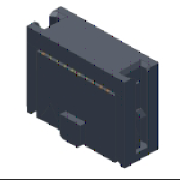
# Autodesk Inventor part: Ribbon Cable Connector-02
Saved by Autodesk Inventor 2017 (Build 210142000, 142)
## iProperties
Created: 2016-02-22
Part Number: Ribbon Cable Connector-02
Material: Generic
Description: 2.54mm (0.10in) Pitch, Receptacle, Vertical, Dual Row
Document SubType Name: Modeling
Designer: qupec
Language: en-US
Size Designation: Ribbon Cable Connector-01
Categories: <MemberInstance><Categories><Category DisplayName="Cable &amp; Harness" InternalName="e4a7e005-5e42-4d16-b293-125e7f0d0512" Mnemonic="CABLEANDHARNESS"><Category DisplayName="Connectors" InternalName="6f634eba-a678-4820-a31d-2c2d5ee6728e" Mnemonic="CONNECTORS"><CategoryParameter DisplayName="RefDes" InternalName="c3740e8c-60ab-4d5d-8584-52b73222f2f0" Mnemonic="REFDES"/><Category DisplayName="Ribbon Cable" InternalName="27621a3d-53ec-49ed-8225-e2ac65e8eb52" Mnemonic="RIBBONCABLE"/></Category></Category><Category DisplayName="DataType" InternalName="23b78d0f-2648-40c6-8793-ca6db495c9e8" Mnemonic="DATATYPE"><CategoryParameter DisplayName="DisplayName" InternalName="05415f3d-3907-474b-a020-eb9d644f4cf3" Mnemonic="DISPLAYNAME"/><CategoryParameter DisplayName="Standard" InternalName="0c0a119c-1e12-4c84-803f-101930972f5e" Mnemonic="STANDARD"/><CategoryParameter DisplayName="Description" InternalName="13903e3d-64b1-4950-80da-f627842ea37f" Mnemonic="DESCRIPTION"/><CategoryParameter DisplayName="Designation" InternalName="2675968c-4ce5-49e0-a4f5-552d29089031" Mnemonic="DESIGNATION"/><CategoryParameter DisplayName="Default Row" InternalName="2af9ec52-faaa-4026-b378-f9fa4afca842" Mnemonic="DEFAULTROW"/><CategoryParameter DisplayName="Folder Name" InternalName="3f06958e-8713-4116-9be7-ed6184ecc97b" Mnemonic="FOLDERNAME"/><CategoryParameter DisplayName="Revision Guid" InternalName="45a75005-10b1-4dfc-8d6d-dfe629f0b93c" Mnemonic="REVISIONGUID"/><CategoryParameter DisplayName="FileName" InternalName="8b46a4cc-9585-4fed-90c3-899f57e09a73" Mnemonic="FILENAME"/><CategoryParameter DisplayName="StdsOrg" InternalName="8f5914e1-4693-403f-8ab5-d37768198c9d" Mnemonic="STDSORG"/><CategoryParameter DisplayName="Family Version" InternalName="914462f6-6e19-4b14-ba84-155b9680b1d0" Mnemonic="FAMILYREVISION"/><CategoryParameter DisplayName="Standard Revision" InternalName="91d5a463-65c2-4fde-b823-3b7fea5e8e17" Mnemonic="STANDARDREVISION"/><CategoryParameter DisplayName="Member Revision" InternalName="a65d44b9-392f-4f4f-857b-e4b3d54996fe" Mnemonic="MEMBERREVISION"/><CategoryParameter DisplayName="ClipFormat" InternalName="bc51e27b-3422-4e78-93ef-cec197ddf230" Mnemonic="CLIPFORMAT"/><CategoryParameter DisplayName="Manufacturer" InternalName="cd6c7a72-a28a-4e50-99a9-2c7f4e13e5ad" Mnemonic="MANUFACTURER"/><CategoryParameter DisplayName="InternalName" InternalName="cf1d0246-76d9-4b4a-8305-fa0409afb5c1" Mnemonic="INTERNALNAME"/><CategoryParameter DisplayName="IsMetric" InternalName="e2385c5b-1ea4-4823-96a8-8de651266ec3" Mnemonic="ISMETRIC"/><Category DisplayName="Part" InternalName="c0e0b642-3bcb-4cc8-9e80-f96d35c4afa4" Mnemonic="PART"><CategoryParameter DisplayName="Part Number" InternalName="016b6077-bfbe-49bd-92c9-d8d59c39c941" Mnemonic="PARTNUMBER"/><CategoryParameter DisplayName="Stock Number" InternalName="4dba7c1c-e26c-444e-836c-b08b433409a8" Mnemonic="STOCKNUMBER"/><CategoryParameter DisplayName="Material Key" InternalName="5c9a8adb-dd2b-4535-b97f-0a94a95fe41f" Mnemonic="MATERIALKEY"/><CategoryParameter DisplayName="Material" InternalName="818a152a-d3c3-49ca-80ee-df7d91421b8e" Mnemonic="MATERIAL"/></Category></Category></Categories><FamilyTemplate Id="Ribbon Cable Connector"><FamilyTemplateParameters><FamilyTemplateParameter ObjectType="kUserParameterObject" ValueType="xs:double" Id="1" ObjectReferenceKey="Circuits"/><FamilyTemplateParameter ObjectType="kUserParameterObject" ValueType="xs:double" Id="2" ObjectReferenceKey="DimA"/><FamilyTemplateParameter ObjectType="kUserParameterObject" ValueType="xs:double" Id="3" ObjectReferenceKey="DimB"/><FamilyTemplateParameter ObjectType="kPropertyObject" ValueType="xs:string" Id="100" ObjectReferenceKey="{32853F0F-3444-11d1-9E93-0060B03C1CA6}" SubObjectId="52"/><FamilyTemplateParameter ObjectType="kPropertyObject" ValueType="xs:string" Id="105" ObjectReferenceKey="{32853F0F-3444-11d1-9E93-0060B03C1CA6}" SubObjectId="5"/><FamilyTemplateParameter ObjectType="kPartComponentDefinitionObject" ValueType="xs:string" Id="110" SubObjectId="Material"/><FamilyTemplateParameter ObjectType="kPartFeatureObject" ValueType="xs:boolean" Id="200" ObjectReferenceKey="1002000010000000700a0100000000008000000000000000" SubObjectId="Suppressed"/><FamilyTemplateParameter ObjectType="kPartFeatureObject" ValueType="xs:boolean" Id="201" ObjectReferenceKey="1002000010000000320b0100000000008000000000000000" SubObjectId="Suppressed"/><FamilyTemplateParameter ObjectType="kPartFeatureObject" ValueType="xs:boolean" Id="202" ObjectReferenceKey="100200001000000044680200000000008000000000000000" SubObjectId="Suppressed"/><FamilyTemplateParameter ObjectType="kPartFeatureObject" ValueType="xs:boolean" Id="203" ObjectReferenceKey="100200001000000061680200000000008000000000000000" SubObjectId="Suppressed"/><FamilyTemplateParameter ObjectType="kPartFeatureObject" ValueType="xs:boolean" Id="204" ObjectReferenceKey="100200001000000064680200000000008000000000000000" SubObjectId="Suppressed"/><FamilyTemplateParameter ObjectType="kPartFeatureObject" ValueType="xs:boolean" Id="205" ObjectReferenceKey="100200001000000067680200000000008000000000000000" SubObjectId="Suppressed"/><FamilyTemplateParameter ObjectType="kPartFeatureObject" ValueType="xs:boolean" Id="206" ObjectReferenceKey="10020000100000006a680200000000008000000000000000" SubObjectId="Suppressed"/><FamilyTemplateParameter ObjectType="kPartFeatureObject" ValueType="xs:boolean" Id="207" ObjectReferenceKey="10020000100000006d680200000000008000000000000000" SubObjectId="Suppressed"/><FamilyTemplateParameter ObjectType="kPartFeatureObject" ValueType="xs:boolean" Id="208" ObjectReferenceKey="100200001000000070680200000000008000000000000000" SubObjectId="Suppressed"/><FamilyTemplateParameter ObjectType="kPartFeatureObject" ValueType="xs:boolean" Id="209" ObjectReferenceKey="100200001000000073680200000000008000000000000000" SubObjectId="Suppressed"/><FamilyTemplateParameter ObjectType="kPartFeatureObject" ValueType="xs:boolean" Id="210" ObjectReferenceKey="100200001000000076680200000000008000000000000000" SubObjectId="Suppressed"/><FamilyTemplateParameter ObjectType="kPartFeatureObject" ValueType="xs:boolean" Id="211" ObjectReferenceKey="100200001000000079680200000000008000000000000000" SubObjectId="Suppressed"/><FamilyTemplateParameter ObjectType="kPartFeatureObject" ValueType="xs:boolean" Id="212" ObjectReferenceKey="10020000100000007c680200000000008000000000000000" SubObjectId="Suppressed"/><FamilyTemplateParameter ObjectType="kPartFeatureObject" ValueType="xs:boolean" Id="213" ObjectReferenceKey="100200001000000047680200000000008000000000000000" SubObjectId="Suppressed"/><FamilyTemplateParameter ObjectType="kPartFeatureObject" ValueType="xs:boolean" Id="214" ObjectReferenceKey="10020000100000007f680200000000008000000000000000" SubObjectId="Suppressed"/><FamilyTemplateParameter ObjectType="kPartFeatureObject" ValueType="xs:boolean" Id="215" ObjectReferenceKey="100200001000000082680200000000008000000000000000" SubObjectId="Suppressed"/><FamilyTemplateParameter ObjectType="kPartFeatureObject" ValueType="xs:boolean" Id="216" ObjectReferenceKey="100200001000000085680200000000008000000000000000" SubObjectId="Suppressed"/><FamilyTemplateParameter ObjectType="kPartFeatureObject" ValueType="xs:boolean" Id="217" ObjectReferenceKey="100200001000000088680200000000008000000000000000" SubObjectId="Suppressed"/><FamilyTemplateParameter ObjectType="kPartFeatureObject" ValueType="xs:boolean" Id="218" ObjectReferenceKey="10020000100000008b680200000000008000000000000000" SubObjectId="Suppressed"/><FamilyTemplateParameter ObjectType="kPartFeatureObject" ValueType="xs:boolean" Id="219" ObjectReferenceKey="10020000100000008e680200000000008000000000000000" SubObjectId="Suppressed"/><FamilyTemplateParameter ObjectType="kPartFeatureObject" ValueType="xs:boolean" Id="220" ObjectReferenceKey="100200001000000091680200000000008000000000000000" SubObjectId="Suppressed"/><FamilyTemplateParameter ObjectType="kPartFeatureObject" ValueType="xs:boolean" Id="221" ObjectReferenceKey="100200001000000094680200000000008000000000000000" SubObjectId="Suppressed"/><FamilyTemplateParameter ObjectType="kPartFeatureObject" ValueType="xs:boolean" Id="222" ObjectReferenceKey="100200001000000097680200000000008000000000000000" SubObjectId="Suppressed"/><FamilyTemplateParameter ObjectType="kPartFeatureObject" ValueType="xs:boolean" Id="223" ObjectReferenceKey="10020000100000009a680200000000008000000000000000" SubObjectId="Suppressed"/><FamilyTemplateParameter ObjectType="kPartFeatureObject" ValueType="xs:boolean" Id="224" ObjectReferenceKey="10020000100000004a680200000000008000000000000000" SubObjectId="Suppressed"/><FamilyTemplateParameter ObjectType="kPartFeatureObject" ValueType="xs:boolean" Id="225" ObjectReferenceKey="10020000100000009d680200000000008000000000000000" SubObjectId="Suppressed"/><FamilyTemplateParameter ObjectType="kPartFeatureObject" ValueType="xs:boolean" Id="226" ObjectReferenceKey="1002000010000000a0680200000000008000000000000000" SubObjectId="Suppressed"/><FamilyTemplateParameter ObjectType="kPartFeatureObject" ValueType="xs:boolean" Id="227" ObjectReferenceKey="1002000010000000a3680200000000008000000000000000" SubObjectId="Suppressed"/><FamilyTemplateParameter ObjectType="kPartFeatureObject" ValueType="xs:boolean" Id="228" ObjectReferenceKey="1002000010000000a6680200000000008000000000000000" SubObjectId="Suppressed"/><FamilyTemplateParameter ObjectType="kPartFeatureObject" ValueType="xs:boolean" Id="229" ObjectReferenceKey="1002000010000000a9680200000000008000000000000000" SubObjectId="Suppressed"/><FamilyTemplateParameter ObjectType="kPartFeatureObject" ValueType="xs:boolean" Id="230" ObjectReferenceKey="1002000010000000ac680200000000008000000000000000" SubObjectId="Suppressed"/><FamilyTemplateParameter ObjectType="kPartFeatureObject" ValueType="xs:boolean" Id="231" ObjectReferenceKey="1002000010000000af680200000000008000000000000000" SubObjectId="Suppressed"/><FamilyTemplateParameter ObjectType="kPartFeatureObject" ValueType="xs:boolean" Id="232" ObjectReferenceKey="1002000010000000b2680200000000008000000000000000" SubObjectId="Suppressed"/><FamilyTemplateParameter ObjectType="kPartFeatureObject" ValueType="xs:boolean" Id="233" ObjectReferenceKey="1002000010000000b5680200000000008000000000000000" SubObjectId="Suppressed"/><FamilyTemplateParameter ObjectType="kPartFeatureObject" ValueType="xs:boolean" Id="234" ObjectReferenceKey="1002000010000000b8680200000000008000000000000000" SubObjectId="Suppressed"/><FamilyTemplateParameter ObjectType="kPartFeatureObject" ValueType="xs:boolean" Id="235" ObjectReferenceKey="10020000100000004f680200000000008000000000000000" SubObjectId="Suppressed"/><FamilyTemplateParameter ObjectType="kPartFeatureObject" ValueType="xs:boolean" Id="236" ObjectReferenceKey="1002000010000000bb680200000000008000000000000000" SubObjectId="Suppressed"/><FamilyTemplateParameter ObjectType="kPartFeatureObject" ValueType="xs:boolean" Id="237" ObjectReferenceKey="1002000010000000be680200000000008000000000000000" SubObjectId="Suppressed"/><FamilyTemplateParameter ObjectType="kPartFeatureObject" ValueType="xs:boolean" Id="238" ObjectReferenceKey="1002000010000000c1680200000000008000000000000000" SubObjectId="Suppressed"/><FamilyTemplateParameter ObjectType="kPartFeatureObject" ValueType="xs:boolean" Id="239" ObjectReferenceKey="1002000010000000c4680200000000008000000000000000" SubObjectId="Suppressed"/><FamilyTemplateParameter ObjectType="kPartFeatureObject" ValueType="xs:boolean" Id="240" ObjectReferenceKey="1002000010000000c7680200000000008000000000000000" SubObjectId="Suppressed"/><FamilyTemplateParameter ObjectType="kPartFeatureObject" ValueType="xs:boolean" Id="241" ObjectReferenceKey="1002000010000000ca680200000000008000000000000000" SubObjectId="Suppressed"/><FamilyTemplateParameter ObjectType="kPartFeatureObject" ValueType="xs:boolean" Id="242" ObjectReferenceKey="1002000010000000cd680200000000008000000000000000" SubObjectId="Suppressed"/><FamilyTemplateParameter ObjectType="kPartFeatureObject" ValueType="xs:boolean" Id="243" ObjectReferenceKey="1002000010000000d0680200000000008000000000000000" SubObjectId="Suppressed"/><FamilyTemplateParameter ObjectType="kPartFeatureObject" ValueType="xs:boolean" Id="244" ObjectReferenceKey="1002000010000000d3680200000000008000000000000000" SubObjectId="Suppressed"/><FamilyTemplateParameter ObjectType="kPartFeatureObject" ValueType="xs:boolean" Id="245" ObjectReferenceKey="1002000010000000d6680200000000008000000000000000" SubObjectId="Suppressed"/><FamilyTemplateParameter ObjectType="kPartFeatureObject" ValueType="xs:boolean" Id="246" ObjectReferenceKey="100200001000000052680200000000008000000000000000" SubObjectId="Suppressed"/><FamilyTemplateParameter ObjectType="kPartFeatureObject" ValueType="xs:boolean" Id="247" ObjectReferenceKey="1002000010000000d9680200000000008000000000000000" SubObjectId="Suppressed"/><FamilyTemplateParameter ObjectType="kPartFeatureObject" ValueType="xs:boolean" Id="248" ObjectReferenceKey="1002000010000000dc680200000000008000000000000000" SubObjectId="Suppressed"/><FamilyTemplateParameter ObjectType="kPartFeatureObject" ValueType="xs:boolean" Id="249" ObjectReferenceKey="1002000010000000df680200000000008000000000000000" SubObjectId="Suppressed"/><FamilyTemplateParameter ObjectType="kPartFeatureObject" ValueType="xs:boolean" Id="250" ObjectReferenceKey="1002000010000000e2680200000000008000000000000000" SubObjectId="Suppressed"/><FamilyTemplateParameter ObjectType="kPartFeatureObject" ValueType="xs:boolean" Id="251" ObjectReferenceKey="1002000010000000e5680200000000008000000000000000" SubObjectId="Suppressed"/><FamilyTemplateParameter ObjectType="kPartFeatureObject" ValueType="xs:boolean" Id="252" ObjectReferenceKey="1002000010000000e8680200000000008000000000000000" SubObjectId="Suppressed"/><FamilyTemplateParameter ObjectType="kPartFeatureObject" ValueType="xs:boolean" Id="253" ObjectReferenceKey="1002000010000000eb680200000000008000000000000000" SubObjectId="Suppressed"/><FamilyTemplateParameter ObjectType="kPartFeatureObject" ValueType="xs:boolean" Id="254" ObjectReferenceKey="1002000010000000ee680200000000008000000000000000" SubObjectId="Suppressed"/><FamilyTemplateParameter ObjectType="kPartFeatureObject" ValueType="xs:boolean" Id="255" ObjectReferenceKey="1002000010000000f1680200000000008000000000000000" SubObjectId="Suppressed"/><FamilyTemplateParameter ObjectType="kPartFeatureObject" ValueType="xs:boolean" Id="256" ObjectReferenceKey="1002000010000000f4680200000000008000000000000000" SubObjectId="Suppressed"/><FamilyTemplateParameter ObjectType="kPartFeatureObject" ValueType="xs:boolean" Id="257" ObjectReferenceKey="100200001000000055680200000000008000000000000000" SubObjectId="Suppressed"/><FamilyTemplateParameter ObjectType="kPartFeatureObject" ValueType="xs:boolean" Id="258" ObjectReferenceKey="1002000010000000f7680200000000008000000000000000" SubObjectId="Suppressed"/><FamilyTemplateParameter ObjectType="kPartFeatureObject" ValueType="xs:boolean" Id="259" ObjectReferenceKey="1002000010000000fa680200000000008000000000000000" SubObjectId="Suppressed"/><FamilyTemplateParameter ObjectType="kPartFeatureObject" ValueType="xs:boolean" Id="260" ObjectReferenceKey="1002000010000000fd680200000000008000000000000000" SubObjectId="Suppressed"/><FamilyTemplateParameter ObjectType="kPartFeatureObject" ValueType="xs:boolean" Id="261" ObjectReferenceKey="100200001000000000690200000000008000000000000000" SubObjectId="Suppressed"/><FamilyTemplateParameter ObjectType="kPartFeatureObject" ValueType="xs:boolean" Id="262" ObjectReferenceKey="100200001000000003690200000000008000000000000000" SubObjectId="Suppressed"/><FamilyTemplateParameter ObjectType="kPartFeatureObject" ValueType="xs:boolean" Id="263" ObjectReferenceKey="100200001000000058680200000000008000000000000000" SubObjectId="Suppressed"/><FamilyTemplateParameter ObjectType="kPartFeatureObject" ValueType="xs:boolean" Id="264" ObjectReferenceKey="10020000100000005b680200000000008000000000000000" SubObjectId="Suppressed"/><FamilyTemplateParameter ObjectType="kPartFeatureObject" ValueType="xs:boolean" Id="265" ObjectReferenceKey="10020000100000005e680200000000008000000000000000" SubObjectId="Suppressed"/></FamilyTemplateParameters></FamilyTemplate><CategoryParameterMap><ParamToTemplateMap><ParamToTemplate CategoryParameter="//CategoryParameter[@InternalName='05415f3d-3907-474b-a020-eb9d644f4cf3']" ConstantValue="Ribbon Cable Connector"/><ParamToTemplate CategoryParameter="//CategoryParameter[@InternalName='0c0a119c-1e12-4c84-803f-101930972f5e']" TemplateParameter="102"/><ParamToTemplate CategoryParameter="//CategoryParameter[@InternalName='13903e3d-64b1-4950-80da-f627842ea37f']" ConstantValue="2.54mm (0.10in) Pitch, Receptacle, Vertical, Dual Row"/><ParamToTemplate CategoryParameter="//CategoryParameter[@InternalName='2af9ec52-faaa-4026-b378-f9fa4afca842']" ConstantValue="1"/><ParamToTemplate CategoryParameter="//CategoryParameter[@InternalName='3f06958e-8713-4116-9be7-ed6184ecc97b']" ConstantValue="Ribbon Cable Connector"/><ParamToTemplate CategoryParameter="//CategoryParameter[@InternalName='45a75005-10b1-4dfc-8d6d-dfe629f0b93c']" ConstantValue="a3a57e36-970e-4b53-b58b-44e930e7e04d"/><ParamToTemplate CategoryParameter="//CategoryParameter[@InternalName='8f5914e1-4693-403f-8ab5-d37768198c9d']" TemplateParameter="101"/><ParamToTemplate CategoryParameter="//CategoryParameter[@InternalName='914462f6-6e19-4b14-ba84-155b9680b1d0']" ConstantValue="11"/><ParamToTemplate CategoryParameter="//CategoryParameter[@InternalName='91d5a463-65c2-4fde-b823-3b7fea5e8e17']" TemplateParameter="103"/><ParamToTemplate CategoryParameter="//CategoryParameter[@InternalName='bc51e27b-3422-4e78-93ef-cec197ddf230']" ConstantValue="CF_INVENTOR.STDPARTS"/><ParamToTemplate CategoryParameter="//CategoryParameter[@InternalName='cd6c7a72-a28a-4e50-99a9-2c7f4e13e5ad']" TemplateParameter="104"/><ParamToTemplate CategoryParameter="//CategoryParameter[@InternalName='cf1d0246-76d9-4b4a-8305-fa0409afb5c1']" ConstantValue="40b76d18-17cd-4eeb-a7c8-2b6dc5bd681a"/><ParamToTemplate CategoryParameter="//CategoryParameter[@InternalName='e2385c5b-1ea4-4823-96a8-8de651266ec3']" ConstantValue="true"/><ParamToTemplate CategoryParameter="//CategoryParameter[@InternalName='8b46a4cc-9585-4fed-90c3-899f57e09a73']" ConstantValue="Ribbon Cable Connector-01"/><ParamToTemplate CategoryParameter="//CategoryParameter[@InternalName='a65d44b9-392f-4f4f-857b-e4b3d54996fe']" ConstantValue="b666cb32-0b43-4429-87d9-31e43f82d377"/><ParamToTemplate CategoryParameter="//CategoryParameter[@InternalName='2675968c-4ce5-49e0-a4f5-552d29089031']" TemplateParameter="100"/><ParamToTemplate CategoryParameter="//CategoryParameter[@InternalName='818a152a-d3c3-49ca-80ee-df7d91421b8e']" TemplateParameter="110"/><ParamToTemplate CategoryParameter="//CategoryParameter[@InternalName='016b6077-bfbe-49bd-92c9-d8d59c39c941']" TemplateParameter="105"/></ParamToTemplateMap></CategoryParameterMap></MemberInstance>
Density: 1 g/cm^3
Appearance: Dark Gray
IsCustomPart: 1
Author: qupec
Autodesk Inventor part; units mm, degrees
ref_plane "YZ Plane" through (0, 0, 0) normal (1, 0, 0) x (0, 1, 0)
ref_plane "XZ Plane" through (0, 0, 0) normal (0, 1, 0) x (-1, 0, 0)
sketch "Sketch1" plane through (0, 0, 0) normal (0, 0, 1) x (1, 0, 0)
  line L0 (-8, -2) -> (8, -2)
  line L1 (8, -2) -> (8, 2)
  line L2 (8, 2) -> (-8, 2)
  line L3 (-8, 2) -> (-8, -2)
  point P0 (0, 0)
  dimension "d268" = 4
  dimension "d269" = 2
  dimension "d270" = 16
  dimension "d271" = 8
  constraints: 8 end point, 2 parallel, 1 horizontal, 1 perpendicular, 1 other
  measures "d268" distance of L2.end L0.start
  measures "d269" distance from line of point (0, 0) L0
  measures "d270" distance between parallel lines of L1 L3
  measures "d271" distance from line of point (0, 0) L3
extrude "Extrusion1" add sketch "Sketch1" along normal blind 10.2
sketch "Sketch2" plane through (-6.98, -2.75, 0) normal (0, -1, 0) x (1, 0, 0)
  line L0 (0, 0) -> (13.96, 0) projected
  line L1 (5.18, 3.6) -> (8.78, 3.6)
  line L2 (8.78, 3.6) -> (8.78, 0.5)
  line L3 (8.28, 0) -> (5.68, 0)
  line L4 (5.18, 0.5) -> (5.18, 3.6)
  line L5 (5.18, 0.5) -> (5.68, 0)
  line L6 (8.78, 0.5) -> (8.28, 0)
  point P0 (6.98, 0)
  dimension "d15" = 3.6
  dimension "d17" = 0.5
  dimension "d19" = 135
  dimension "d20" = 135
  dimension "d21" = 0.5
  dimension "d22" = 3.6
  constraints: 12 end point, 2 midpoint, 2 parallel, 1 horizontal, 1 perpendicular
  measures "d15" distance of L1.start L1.end
  measures "d17" horizontal distance of L3.end L4.start
  measures "d19" angle of L5 L4
  measures "d20" angle of L6 L2
  measures "d21" horizontal distance of L3.start L2.end
  measures "d22" distance between parallel lines of L0 L1
extrude "Extrusion2" [suppressed]
sketch "Sketch3" plane through (0, 0, 0) normal (0, 1, 0) x (-1, 0, 0)
  line L0 (-6.98, 3.6) -> (-7.23, 3.6)
  line L1 (-7.98, 2.1) -> (-7.98, 1.22)
  line L2 (-7.98, 1.22) -> (-6.98, 1.22)
  line L3 (-6.98, 1.22) -> (-6.98, 3.6)
  line L4 (6.98, 10.2) -> (-6.98, 10.2) projected
  line L5 (0, 10.2) -> (0, 0)
  line L6 (-6.98, 0) -> (6.98, 0) projected
  line L7 (-7.23, 3.6) -> (-7.98, 2.1)
  line L8 (6.98, 3.6) -> (7.23, 3.6)
  line L9 (7.98, 2.1) -> (7.98, 1.22)
  line L10 (7.98, 1.22) -> (6.98, 1.22)
  line L11 (6.98, 1.22) -> (6.98, 3.6)
  line L12 (7.23, 3.6) -> (7.98, 2.1)
  dimension "d25" = 13.96
  dimension "d26" = 1.22
  dimension "d28" = 1
  dimension "d29" = 1.5
  dimension "d30" = 0.88
  dimension "d31" = 0.25
  constraints: 22 end point, 5 symmetric about line, 2 midpoint, 2 parallel, 2 perpendicular, 1 horizontal
  measures "d25" diameter of L3 L5
  measures "d26" distance between parallel lines of L2 L6
  measures "d28" distance of L1.end L2.end
  measures "d29" vertical distance of L0.end L1.start
  measures "d30" distance of L1.start L1.end
  measures "d31" distance of L0.start L0.end
extrude "Extrusion3" [suppressed]
sketch "Sketch4" plane through (0, -0.5, 0) normal (0, -1, 0) x (1, 0, 0)
  line L0 (6.98, 3.6) -> (7.23, 3.6) projected
  line L1 (6.98, 6.263) -> (7.23, 6.263)
  line L2 (7.98, 5.513) -> (7.98, 5.263)
  line L3 (7.98, 5.263) -> (6.98, 5.263)
  line L4 (6.98, 5.263) -> (6.98, 6.263)
  line L5 (-6.98, 10.2) -> (6.98, 10.2) projected
  line L6 (6.98, 0) -> (-6.98, 0) projected
  line L7 (0, 10.2) -> (0, 0)
  line L8 (7.23, 6.263) -> (7.98, 5.513)
  line L9 (-6.98, 6.263) -> (-7.23, 6.263)
  line L10 (-7.98, 5.513) -> (-7.98, 5.263)
  line L11 (-7.98, 5.263) -> (-6.98, 5.263)
  line L12 (-6.98, 5.263) -> (-6.98, 6.263)
  line L13 (-7.23, 6.263) -> (-7.98, 5.513)
  dimension "d34" = 1.663
  dimension "d35" = 13.96
  dimension "d36" = 1
  dimension "d38" = 0.25
  dimension "d39" = 1
  dimension "d40" = 0.25
  constraints: 22 end point, 5 symmetric about line, 2 midpoint, 2 parallel, 1 horizontal, 1 perpendicular
  measures "d34" distance between parallel lines of L3 L0
  measures "d35" diameter of L4 L7
  measures "d36" distance of L2.end L3.end
  measures "d38" distance of L1.start L1.end
  measures "d39" distance of L3.end L1.start
  measures "d40" distance of L2.start L2.end
extrude "Extrusion4" [suppressed]
sketch "Sketch5" plane through (0, 0.5, 0) normal (0, 1, 0) x (1, 0, 0)
  line L0 (7.23, -3.6) -> (6.98, -3.6) projected
  line L1 (7.23, -6.263) -> (6.98, -6.263)
  line L2 (6.98, -6.263) -> (6.98, -5.263)
  line L3 (6.98, -5.263) -> (7.98, -5.263)
  line L4 (7.98, -5.263) -> (7.98, -5.513)
  line L5 (6.98, -10.2) -> (-6.98, -10.2) projected
  line L6 (1.3, 0) -> (-1.3, 0) projected
  line L7 (0, 0) -> (0, -10.2)
  line L8 (7.23, -6.263) -> (7.98, -5.513)
  line L9 (-7.23, -6.263) -> (-6.98, -6.263)
  line L10 (-6.98, -6.263) -> (-6.98, -5.263)
  line L11 (-6.98, -5.263) -> (-7.98, -5.263)
  line L12 (-7.98, -5.263) -> (-7.98, -5.513)
  line L13 (-7.23, -6.263) -> (-7.98, -5.513)
  dimension "d43" = 1.663
  dimension "d44" = 13.96
  dimension "d45" = 1
  dimension "d46" = 1
  dimension "d47" = 0.25
  dimension "d48" = 0.25
  constraints: 22 end point, 5 symmetric about line, 2 midpoint, 2 parallel, 1 horizontal, 1 perpendicular
  measures "d43" distance between parallel lines of L0 L3
  measures "d44" diameter of L2 L7
  measures "d45" distance of L1.end L2.end
  measures "d46" distance of L2.end L3.end
  measures "d47" distance of L1.start L1.end
  measures "d48" distance of L3.end L4.end
extrude "Extrusion5" [suppressed]
sketch "Sketch6" plane through (-6.98, -2.75, 10.2) normal (0, -1, 0) x (1, 0, 0)
  line L0 (0, -10.2) -> (5.68, -10.2) projected
  line L1 (-38.97, -10.2) -> (-36.97, -6.7359)
  line L2 (-36.97, -6.7359) -> (-34.97, -10.2)
  line L3 (-38.97, -10.2) -> (-34.97, -10.2)
  line L4 (0.5, -10.2) -> (2.5, -6.7359)
  line L5 (2.5, -6.7359) -> (4.5, -10.2)
  line L6 (0.5, -10.2) -> (4.5, -10.2)
  dimension "d61" = 0.5
  dimension "d62" = 4
  constraints: 12 end point, 4 equal length, 2 point on line, 1 collinear
  measures "d61" distance of L4.start L0.start
  measures "d62" distance of L4.start L5.end
extrude "Extrusion6" [suppressed]
sketch "Sketch7" plane through (0, 0, 0) normal (0, 0, -1) x (-1, 0, 0)
  line L0 (6.98, 2.75) -> (6.98, -1.25) projected
  line L1 (4.705, 1.645) -> (5.455, 1.645)
  line L2 (5.455, 1.645) -> (5.455, 0.895)
  line L3 (5.455, 0.895) -> (4.705, 0.895)
  line L4 (4.705, 0.895) -> (4.705, 1.645)
  line L5 (4.705, -0.895) -> (5.455, -0.895)
  line L6 (5.455, -0.895) -> (5.455, -1.645)
  line L7 (5.455, -1.645) -> (4.705, -1.645)
  line L8 (4.705, -1.645) -> (4.705, -0.895)
  line L9 (5.08, 0.895) -> (5.08, -0.895) construction
  point P0 (0, 0)
  point P1 (5.08, 0)
  dimension "d65" = 0.75
  dimension "d66" = 2.54
  dimension "d67" = 1.525
  constraints: 18 end point, 7 equal length, 4 parallel, 3 midpoint, 3 perpendicular, 2 horizontal, 1 horizontal alignment
  measures "d65" distance of L1.start L1.end
  measures "d66" distance between parallel lines of L5 L1
  measures "d67" distance between parallel lines of L0 L6
extrude "Extrusion7" [suppressed]
chamfer "Chamfer1" [suppressed]
pattern_linear "Rectangular Pattern1" [suppressed]
ref_plane "Work Plane1" through (0, 0, 10.7) normal (0, 0, 1) x (1, 0, 0)
sketch "Sketch8" plane through (0, 0, 10.7) normal (0, 0, 1) x (1, 0, 0)
  line L0 (-6.98, 2.75) -> (6.98, 2.75) projected
  line L1 (-6.98, -2.75) -> (-6.98, 2.75) projected
  line L2 (6.98, -2.75) -> (-6.98, -2.75) projected
  line L3 (6.98, 2.75) -> (6.98, -2.75) projected
  line L4 (-7.11, 0) -> (-42.9538, 0)
  line L5 (-8, -2) -> (-8, 2) projected
  line L6 (8, -2) -> (-8, -2) projected
  line L7 (8, 2) -> (8, -2) projected
  line L8 (-8, 2) -> (8, 2) projected
  line L9 (8, 2) -> (-8, 2) projected
  line L10 (8, -2) -> (-8, -2)
  line L11 (-8, -2) -> (-8, 2)
  line L12 (-8, 2) -> (8, 2)
  line L13 (8, 2) -> (8, -2)
  constraints: 10 end point, 2 parallel, 1 horizontal, 1 perpendicular, 1 other
extrude "Extrusion20" add sketch "Sketch8" along normal blind 0.8 contours L8 L3 L6 L1 | L1 L6 L5 L8 | L8 L7 L6 L3
sketch "Sketch22" plane through (0, 0, 0) normal (0, 0, -1) x (-1, 0, 0)
  line L0 (-7.99, -3) -> (-8.665, -3) projected
  line L1 (8.665, 2.75) -> (-8.665, 2.75) projected
  line L2 (-8.665, -3) -> (8.665, -3)
  line L3 (8.665, -3) -> (8.665, 2.75)
  line L4 (8.665, 2.75) -> (-8.665, 2.75)
  line L5 (-8.665, 2.75) -> (-8.665, -3)
  point P0 (0, 0)
  constraints: 8 end point, 2 parallel, 1 horizontal, 1 perpendicular
extrude "Extrusion17" [suppressed]
sketch "Sketch25" plane through (0, 0, 0) normal (0, 0, -1) x (-1, 0, 0)
  line L0 (8, -2) -> (-8, -2) projected
  line L1 (8, 2) -> (8, -2) projected
  line L2 (-8, 2) -> (8, 2) projected
  line L3 (-8, -2) -> (-8, 2) projected
  line L4 (8, -2) -> (-8, -2)
  line L5 (-8, -2) -> (-8, 2)
  line L6 (-8, 2) -> (8, 2)
  line L7 (8, 2) -> (8, -2)
  point P0 (0, 0)
  constraints: 8 end point, 2 parallel, 1 horizontal, 1 perpendicular
extrude "Extrusion21" cut sketch "Sketch25" against normal blind 9.1
sketch "Sketch26" plane through (0, 0, 10.2) normal (0, 0, 1) x (1, 0, 0)
  line L0 (8, -2) -> (-8, -2) projected
  line L1 (8, 2) -> (-8, 2) projected
  line L2 (-8, -2) -> (-7, -2)
  line L3 (-7, -2) -> (-7, 2)
  line L4 (-7, 2) -> (-8, 2)
  line L5 (-8, 2) -> (-8, -2)
  point P0 (0, 0)
  dimension "d276" = 1
  constraints: 8 end point, 2 parallel, 1 horizontal, 1 perpendicular, 1 point on line
  measures "d276" distance between parallel lines of L5 L3
extrude "Extrusion22" add sketch "Sketch26" along normal blind 0.5
mirror "Mirror1" about plane through (0, 0, 0) normal (1, 0, 0) of "Extrusion22"
equation "\"DimA\" = 13.96"
equation "\"DimB\" = 17.33"
equation "\"DimC\" = 5.715"
body "Solid1"
